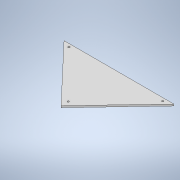
# Autodesk Inventor part: aab_pcb
Saved by Autodesk Inventor 2020 (Build 240168000, 168)
## iProperties
Created: 2019-09-26
Part Number: aab_pcb
Material: Generic
Document SubType Name: Modeling
Designer: fabrizio
Density: 1 g/cm^3
Appearance: Default
Author: fabrizio
Autodesk Inventor part; units mm, degrees
ref_plane "YZ Plane" through (0, 0, 0) normal (1, 0, 0) x (0, 1, 0)
ref_plane "XZ Plane" through (0, 0, 0) normal (0, 1, 0) x (-1, 0, 0)
ref_plane "XY Plane" through (0, 0, 0) normal (0, 0, 1) x (1, 0, 0)
sketch "Sketch1" plane through (0, 0, 0) normal (0, 1, 0) x (-1, 0, 0)
  circle A0 centre (64.0457, 59.1814) radius 1
  circle A1 centre (9.3447, 3.6422) radius 1
  circle A2 centre (118.7247, 3.6422) radius 1
  line L0 (0, 0) -> (128.06, 0)
  line L1 (128.06, 0) -> (64.0431, 67.5178)
  line L2 (64.0431, 67.5178) -> (0, 0)
  constraints: 6 end point, 3 centre point
extrude "Extrusion1" add sketch "Sketch1" along normal blind 2
body "Solid1"
